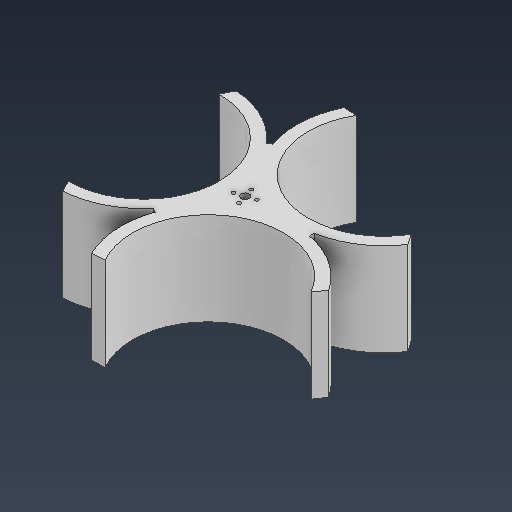
# Autodesk Inventor part: сюрикен 2 dthcbz
Saved by Autodesk Inventor 2026 (Build 300175000, 175)
## iProperties
Created: 2025-11-21
Part Number: сюрикен 2 dthcbz
Material: Типовые
Document SubType Name: Modeling
Designer: Phantom
Density: 1 g/cm^3
Appearance: По умолчанию
Author: Phantom
Autodesk Inventor part; units mm, degrees
ref_plane "YZ Plane" through (0, 0, 0) normal (1, 0, 0) x (0, 1, 0)
ref_plane "XZ Plane" through (0, 0, 0) normal (0, 1, 0) x (-1, 0, 0)
ref_plane "XY Plane" through (0, 0, 0) normal (0, 0, 1) x (1, 0, 0)
sketch "Эскиз1" plane through (0, 0, 0) normal (0, 1, 0) x (-1, 0, 0)
  circle A0 centre (0, 0) radius 152.5
  line L0 (0, 0) -> (152.5, 0)
  circle A1 centre (87.5, 0) radius 65
  circle A2 centre (-43.75, 75.7772) radius 65
  circle A3 centre (-43.75, -75.7772) radius 65
  circle A4 centre (87.5, 0) radius 75
  circle A5 centre (-43.75, 75.7772) radius 75
  circle A6 centre (-43.75, -75.7772) radius 75
  line L1 (0, 0) -> (-76.25, 132.0689)
  line L2 (0, 0) -> (-76.25, -132.0689)
  line L3 (144.5, 48.7442) -> (30.5, -48.7442)
  line L4 (-114.4637, 100.7686) -> (26.9637, 50.7859)
  line L5 (-30.0363, -149.5128) -> (-57.4637, -2.0417)
  line L6 (30.5, -48.7442) -> (26.9637, -50.7859)
  line L7 (26.9637, 50.7859) -> (30.5, 48.7442)
  line L8 (-57.4637, -2.0417) -> (-57.4637, 2.0417)
  line L9 (87.5, -75) -> (87.5, 75)
  line L10 (21.2019, 113.2772) -> (-108.7019, 38.2772)
  line L11 (-108.7019, -38.2772) -> (21.2019, -113.2772)
  point P0 (14.0693, 24.3687)
  point P1 (-28.1386, 0)
  point P2 (14.0693, -24.3687)
  point P3 (12.5, 0)
  point P4 (22.5, 0)
  point P5 (152.5, 0)
  point P6 (-6.25, 10.8253)
  point P7 (-11.25, 19.4856)
  point P8 (-76.25, 132.0689)
  point P9 (-114.4637, 100.7686)
  point P10 (-6.25, -10.8253)
  point P11 (-11.25, -19.4856)
  point P12 (-76.25, -132.0689)
  point P13 (-30.0363, -149.5128)
  point P14 (-114.4637, -100.7686)
  point P15 (-30.0363, 149.5128)
  point P16 (144.5, -48.7442)
  point P17 (152.5, 0)
  point P18 (136.9, 42.245)
  point P19 (17.5352, 54.1181)
  point P20 (-105.0352, 97.4364)
  point P21 (-114.4637, 100.7686)
  point P22 (-57.4637, -2.0417)
  point P23 (-55.6352, -11.8731)
  point P24 (-31.8648, -139.6814)
  point P25 (-30.0363, -149.5128)
  point P26 (38.1, -42.245)
  point P27 (87.5, -65)
  point P28 (87.5, 65)
  point P29 (12.5417, 108.2772)
  point P30 (-100.0417, 43.2772)
  point P31 (-57.4637, -2.0417)
  point P32 (-100.0417, -43.2772)
  point P33 (12.5417, -108.2772)
  dimension "d0" = 305
  dimension "d1" = 130
  dimension "d2" = 0
  dimension "d5" = 360
  dimension "d7" = 150
  dimension "d10" = 360
  dimension "d16" = 360
  dimension "d18" = 0
  dimension "d21" = 360
  dimension "d25" = 360
  dimension "d48" = 360
  constraints: 24 end point, 6 centre point, 6 point on circle, 4 coincident, 1 horizontal, 1 tangent, 1 vertical, 58 other
  measures "d0" diameter of A0
  measures "d1" diameter of A1
  measures "d2" distance from line of L0 A1.centre
  measures "d7" diameter of A4
  measures "d18" distance from line of A1.centre L3
extrude "Выдавливание1" add sketch "Эскиз1" along normal blind 80 contours L9 A4 L3 A1 | L9 A1 L0 A4 | A1 L3 A4 L0 | A5 L4 A2 L10 | A4 L0 L1 A5 L7 | L11 A3 L2 A6 | L6 A6 L2 L0 A4 | L10 A2 L1 A5 | A5 L1 A2 L4 | L11 A6 L5 A3 | L2 A6 L8 A5 L1 | L5 A6 L2 A3 picked at (58.9785, -61.9188) picked at (22.0957, 93.4205) picked at (-83.1125, -20.1174)
sketch "Эскиз4" plane through (0, 80, 0) normal (0, 1, 0) x (1, 0, 0)
  circle A0 centre (0, 0) radius 3.5
  dimension "d43" = 7
  constraints: 1 centre point, 1 coincident
  measures "d43" diameter of A0
extrude "Выдавливание4" cut sketch "Эскиз4" against normal blind 140
sketch "Эскиз5" plane through (0, 80, 0) normal (0, 1, 0) x (1, 0, 0)
  circle A0 centre (0, 0) radius 3.5 projected
  arc A1 (-87.5, -65) -> (-87.5, 65) centre (-87.5, 0) ccw projected
  line L0 (-87.5, -65) -> (-87.5, -69)
  line L1 (-87.5, -65) -> (-87.5, -75) projected
  circle A2 centre (0, 0) radius 111.4327
  circle A3 centre (0, 0) radius 192.7389
  dimension "d51" = 4
  constraints: 2 coincident, 2 end point, 1 centre point, 1 point on line, 3 other
  measures "d51" distance of L0.start L0.end
extrude "Выдавливание5" cut sketch "Эскиз5" against normal through all contours A3
sketch "Эскиз6" plane through (0, 80, 0) normal (0, 1, 0) x (1, 0, 0)
  line L0 (103.5058, 41.2772) -> (100.0417, 43.2772) projected
  arc A0 (57.4637, 2.0417) -> (106.0924, 34.0829) centre (43.75, 75.7772) ccw projected
  line L1 (100.0417, 43.2772) -> (106.0924, 34.0829)
  line L2 (-87.5, 65) -> (-82.5629, 74.8373)
  line L3 (-12.5417, -108.2772) -> (-23.5296, -108.9202)
  line L4 (100.0417, -43.2772) -> (103.5058, -41.2772) projected
  line L5 (106.0924, -34.0829) -> (100.0417, -43.2772)
  line L6 (-23.5296, 108.9202) -> (-12.5417, 108.2772)
  line L7 (-82.5629, -74.8373) -> (-87.5, -65)
  arc A1 (-12.5417, 108.2772) -> (100.0417, 43.2772) centre (43.75, 75.7772) ccw projected
  arc A2 (-82.5629, 74.8373) -> (-87.5, 69) centre (0, 0) ccw projected
  line L8 (-87.5, 69) -> (-87.5, 65) projected
  arc A3 (-87.5, -65) -> (-87.5, 65) centre (-87.5, 0) ccw projected
  line L9 (-87.5, -65) -> (-87.5, -69) projected
  arc A4 (-87.5, -69) -> (-82.5629, -74.8373) centre (0, 0) ccw projected
  arc A5 (-82.5629, -74.8373) -> (-30.5, -48.7442) centre (-87.5, 0) ccw projected
  line L10 (-30.5, -48.7442) -> (-26.9637, -50.7859) projected
  arc A6 (-26.9637, -50.7859) -> (-23.5296, -108.9202) centre (43.75, -75.7772) ccw projected
  arc A7 (-23.5296, -108.9202) -> (-16.0058, -110.2772) centre (0, 0) ccw projected
  line L11 (-16.0058, -110.2772) -> (-12.5417, -108.2772) projected
  arc A8 (100.0417, -43.2772) -> (-12.5417, -108.2772) centre (43.75, -75.7772) ccw projected
  line L12 (100.0417, -43.2772) -> (103.5058, -41.2772) projected
  arc A9 (103.5058, -41.2772) -> (106.0924, -34.0829) centre (0, 0) ccw projected
  arc A10 (106.0924, -34.0829) -> (57.4637, -2.0417) centre (43.75, -75.7772) ccw projected
  line L13 (57.4637, -2.0417) -> (57.4637, 2.0417) projected
  arc A11 (57.4637, 2.0417) -> (106.0924, 34.0829) centre (43.75, 75.7772) ccw projected
  arc A12 (106.0924, 34.0829) -> (103.5058, 41.2772) centre (0, 0) ccw projected
  line L14 (103.5058, 41.2772) -> (100.0417, 43.2772) projected
  arc A13 (-12.5417, 108.2772) -> (100.0417, 43.2772) centre (43.75, 75.7772) ccw projected
  line L15 (-12.5417, 108.2772) -> (-16.0058, 110.2772) projected
  arc A14 (-16.0058, 110.2772) -> (-23.5296, 108.9202) centre (0, 0) ccw projected
  arc A15 (-23.5296, 108.9202) -> (-26.9637, 50.7859) centre (43.75, 75.7772) ccw projected
  line L16 (-26.9637, 50.7859) -> (-30.5, 48.7442) projected
  arc A16 (-30.5, 48.7442) -> (-82.5629, 74.8373) centre (-87.5, 0) ccw projected
  circle A17 centre (0, 0) radius 3.5 projected
  point P0 (-12.5417, 108.2772)
  point P1 (106.0924, 34.0829)
  dimension "d56" = 360
  dimension "d60" = 360
  constraints: 12 end point, 20 other
extrude "Выдавливание6" cut sketch "Эскиз6" against normal through all contours A12 L1 L0 | L6 A14 L15 | A9 L4 L5 | L2 L8 A2 | L11 A7 L3 | L7 A4 L9
sketch "Эскиз7" plane through (0, 80, 0) normal (0, 1, 0) x (1, 0, 0)
  circle A0 centre (7.6092, 2.4699) radius 1.6
  circle A1 centre (-7.6092, -2.4699) radius 1.6
  circle A2 centre (-2.4699, 7.6092) radius 1.6
  circle A3 centre (0, 0) radius 3.1
  circle A4 centre (2.4699, -7.6092) radius 1.6
  constraints: 5 centre point
extrude "Выдавливание7" cut sketch "Эскиз7" against normal through all contours A0 | A1 | A2 | A4
